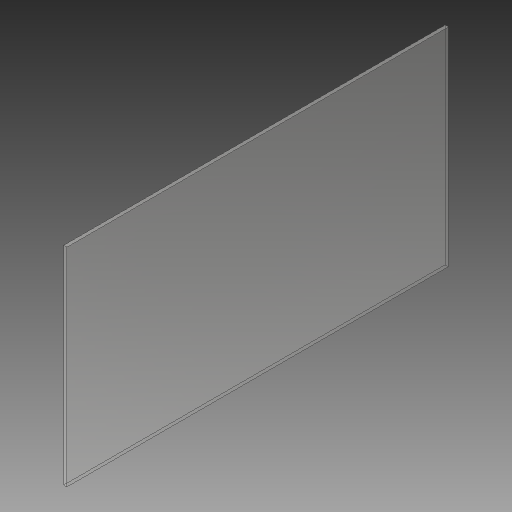
# Autodesk Inventor part: 15102898-16-P-0401
Saved by Autodesk Inventor 2017 (Build 210142000, 142)
## iProperties
Created: 2016-10-03
Part Number: 15102898-16-P-0401
Material: Polycarbonate, Clear
Document SubType Name: Modeling
Designer: gus
Density: 1.2 g/cm^3
Appearance: Polycarbonate - Clear
Mass: 2312.23 g
Surface Area: 6215.28 cm^2
Volume: 1926.86 cm^3
Author: gus
Autodesk Inventor part; units mm, degrees
ref_plane "YZ Plane" through (0, 0, 0) normal (1, 0, 0) x (0, 1, 0)
ref_plane "XZ Plane" through (0, 0, 0) normal (0, 1, 0) x (-1, 0, 0)
ref_plane "XY Plane" through (0, 0, 0) normal (0, 0, 1) x (1, 0, 0)
sketch "Sketch1" plane through (0, 0, 0) normal (1, 0, 0) x (0, 1, 0)
  line L0 (0, 0) -> (406.4, 0)
  line L1 (406.4, 0) -> (406.4, -746.6584)
  line L2 (406.4, -746.6584) -> (0, -746.6584)
  line L3 (0, -746.6584) -> (0, 0)
  dimension "d0" = 406.4
  dimension "d1" = 746.6584
  constraints: 8 end point, 2 parallel, 1 horizontal, 1 perpendicular
  measures "d0" distance of L1.end L2.end
  measures "d1" distance of L0.end L1.end
extrude "Extrusion1" add sketch "Sketch1" along normal blind 6.35
body "Solid1"
